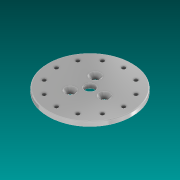
# Autodesk Inventor part: end effector mount 4 mm
Saved by Autodesk Inventor 2020.3 (Build 243373000, 373)
## iProperties
Created: 2020-05-18
Part Number: end effector mount 4 mm
Material: Aluminum 6061
Document SubType Name: Modeling
Designer: stefa
Density: 2.7 g/cm^3
Appearance: Aluminum - Polished
Mass: 36.8552 g
Surface Area: 63.4935 cm^2
Volume: 13.6501 cm^3
Author: stefa
Autodesk Inventor part; units mm, degrees
ref_plane "YZ Plane" through (0, 0, 0) normal (1, 0, 0) x (0, 1, 0)
ref_plane "XZ Plane" through (0, 0, 0) normal (0, 1, 0) x (-1, 0, 0)
ref_plane "XY Plane" through (0, 0, 0) normal (0, 0, 1) x (1, 0, 0)
sketch "Sketch1" plane through (0, 0, 0) normal (0, 1, 0) x (-1, 0, 0)
  circle A0 centre (0, 0) radius 4
  circle A1 centre (0, 0) radius 35
  circle A2 centre (0, -28) radius 2
  circle A3 centre (14, -24.2487) radius 2
  circle A4 centre (24.2487, -14) radius 2
  circle A5 centre (28, 0) radius 2
  circle A6 centre (24.2487, 14) radius 2
  circle A7 centre (14, 24.2487) radius 2
  circle A8 centre (0, 28) radius 2
  circle A9 centre (-14, 24.2487) radius 2
  circle A10 centre (-24.2487, 14) radius 2
  circle A11 centre (-28, 0) radius 2
  circle A12 centre (-24.2487, -14) radius 2
  circle A13 centre (-14, -24.2487) radius 2
  circle A14 centre (-12, 0) radius 2.05
  circle A15 centre (6, -10.3923) radius 2.05
  circle A16 centre (6, 10.3923) radius 2.05
  dimension "d0" = 70
  dimension "d1" = 8
  dimension "d4" = 4
  dimension "d5" = 28
  dimension "d8" = 360
  dimension "d21" = 14.4939
  dimension "d53" = 12
  dimension "d54" = 4.1
  dimension "d57" = 360
  constraints: 17 centre point, 2 coincident, 1 horizontal alignment, 1 vertical alignment, 32 other
  measures "d0" diameter of A1
  measures "d1" diameter of A0
  measures "d4" diameter of A2
  measures "d5" distance of A2.centre point (0, 0)
  measures "d21" distance of A3.centre A4.centre
  measures "d53" distance of point (0, 0) A14.centre
  measures "d54" diameter of A14
extrude "Extrusion1" add sketch "Sketch1" along normal blind 4 contours A1 | A2 | A3 | A4 | A5 | A6 | A7 | A8 | A9 | A10 | A11 | A12 | A13
chamfer "Chamfer2" distance 0.5 angle 45 4 edges at (35, 4, 0) (4, 4, 0) (35, 0, 0) (4, 0, 0)
chamfer "Chamfer3" distance 2.5 angle 45 3 edges at (-3.95, 4, 10.3923) (-3.95, 4, -10.3923) (14.05, 4, 0)
hole "Hole1" at (-24.2487, 0, -14) at (-28, 0, 0) at (-24.2487, 0, 14) at (-14, 0, 24.2487) at (0, 0, 28) at (14, 0, 24.2487) at (24.2487, 0, 14) at (28, 0, 0) at (24.2487, 0, -14) at (14, 0, -24.2487) at (0, 0, -28) at (-14, 0, -24.2487) direction (0, 1, 0) diameter 3.242 depth 15 tip angle 118 thread size "M4x0.7" class "6H" standard "ISO Metric profile"
body "Solid1"
